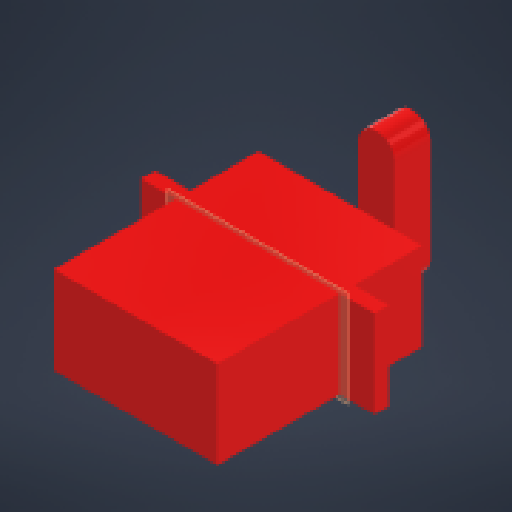
# Autodesk Inventor part: Servo
Saved by Autodesk Inventor 2026 (Build 300175050, 175E)
## iProperties
Created: 2026-02-21
Part Number: Servo
Material: LCP plast
Document SubType Name: Modeling
Designer: marti
Density: 1.626 g/cm^3
Appearance: Hladká – červená
Author: marti
Autodesk Inventor part; units mm, degrees
ref_plane "YZ Plane" through (0, 0, 0) normal (1, 0, 0) x (0, 1, 0)
ref_plane "XZ Plane" through (0, 0, 0) normal (0, 1, 0) x (-1, 0, 0)
sketch "Náčrt1" plane through (0, 0, 0) normal (0, 0, 1) x (1, 0, 0)
  line L0 (-11.4, 6.1) -> (11.4, 6.1)
  line L1 (11.4, 6.1) -> (11.4, -6.1)
  line L2 (11.4, -6.1) -> (-11.4, -6.1)
  line L3 (-11.4, -6.1) -> (-11.4, 6.1)
  line L4 (0, 8.54) -> (0, -8.54) projected
  line L5 (-15.96, 0) -> (15.96, 0) projected
  point P0 (0, 0)
  dimension "d0" = 22.8
  dimension "d1" = 12.2
  constraints: 8 end point, 2 parallel, 1 horizontal, 1 perpendicular, 2 other
  measures "d0" distance of L1.end L2.end
  measures "d1" distance of L0.end L1.end
extrude "Vysunutí1" add sketch "Náčrt1" against normal blind 28.5
ref_plane "Pracovní rovina1" through (0, 0, -17) normal (0, 0, 1) x (1, 0, 0)
sketch "Náčrt2" plane through (0, 0, -17) normal (0, 0, 1) x (1, 0, 0)
  line L0 (11.4, 6.1) -> (11.4, -6.1) projected
  line L1 (11.4, -6.1) -> (-11.4, -6.1) projected
  line L2 (-11.4, -6.1) -> (-11.4, 6.1) projected
  line L3 (-11.4, 6.1) -> (11.4, 6.1) projected
  line L4 (16.25, 6.1) -> (-16.25, 6.1)
  line L5 (-16.25, 6.1) -> (-16.25, -6.1)
  line L6 (-16.25, -6.1) -> (16.25, -6.1)
  line L7 (16.25, -6.1) -> (16.25, 6.1)
  line L8 (-22.75, 0) -> (22.75, 0) projected
  line L9 (0, 8.54) -> (0, -8.54) projected
  point P0 (0, 0)
  dimension "d5" = 32.5
  dimension "d6" = 12.2
  constraints: 8 end point, 2 parallel, 1 horizontal, 1 perpendicular, 2 other
  measures "d5" distance between parallel lines of L5 L7
  measures "d6" distance between parallel lines of L6 L4
extrude "Vysunutí2" add sketch "Náčrt2" against normal blind 2
ref_plane "Pracovní rovina2" through (5, 0, -33.5) normal (0, 0, -1) x (-1, 0, 0)
sketch "Náčrt4" plane through (5, 0, -33.5) normal (0, 0, -1) x (-1, 0, 0)
  circle A0 centre (0, 0) radius 2.5 projected
  circle A1 centre (0, 14.2756) radius 2.5
  line L0 (2.5, 14.2756) -> (2.5, 0)
  line L1 (-26.45, 0) -> (29.2, 0) projected
  line L2 (5, -10.6881) -> (5, 21.4288) projected
  line L3 (-2.5, 14.2756) -> (-2.5, 0)
  point P0 (5, 0)
  dimension "d15" = 90
  dimension "d16" = 2.5
  constraints: 5 point on circle, 4 end point, 2 tangent, 1 centre point, 1 point on line
  measures "d15" angle of L1 L0
  measures "d16" distance from line of L0 A1.centre
extrude "Vysunutí4" add sketch "Náčrt4" against normal blind 5
